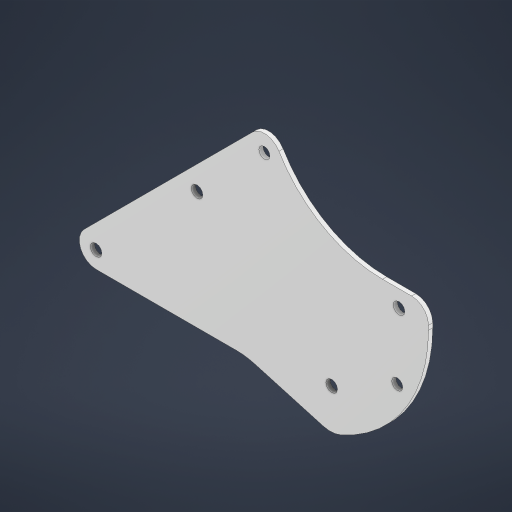
# Autodesk Inventor part: sled
Saved by Autodesk Inventor 2024 (Build 280153000, 153)
## iProperties
Created: 2023-08-16
Part Number: sled
Material: Acetal Resin, White
Document SubType Name: Modeling
Designer: avere
Density: 1.425 g/cm^3
Appearance: Smooth - White
Author: avere
Autodesk Inventor part; units mm, degrees
ref_plane "YZ Plane" through (0, 0, 0) normal (1, 0, 0) x (0, 1, 0)
ref_plane "XZ Plane" through (0, 0, 0) normal (0, 1, 0) x (-1, 0, 0)
ref_plane "XY Plane" through (0, 0, 0) normal (0, 0, 1) x (1, 0, 0)
sketch "Sketch1" plane through (0, 0, 0) normal (0, 0, 1) x (1, 0, 0)
  circle A0 centre (-18.3721, 25.1477) radius 2.1844
  circle A1 centre (57.8279, 25.1477) radius 2.1844
  circle A2 centre (32.4279, -12.9523) radius 2.1844
  circle A3 centre (-56.4721, -12.9523) radius 2.1844
  arc A4 (-60.9623, -8.4622) -> (-56.4721, -19.3023) centre (-56.4721, -12.9523) ccw
  arc A5 (-18.3721, 31.4977) -> (-22.8623, 29.6378) centre (-18.3721, 25.1477) ccw
  line L0 (68.9404, 23.5133) -> (68.9404, 25.1477)
  line L1 (62.5904, 31.4977) -> (57.8279, 31.4977)
  arc A6 (68.9404, 25.1477) -> (62.5904, 31.4977) centre (62.5904, 25.1477) ccw
  line L2 (-3.5614, -19.3023) -> (-56.4721, -19.3023)
  line L3 (-60.9623, -8.4622) -> (-22.8623, 29.6378)
  line L4 (-18.3721, 31.4977) -> (57.8279, 31.4977)
  arc A7 (35.7428, -27.2531) -> (68.9404, 23.5133) centre (13.525, 23.5133) ccw
  line L5 (29.3044, -27.6849) -> (3.4241, -20.2818)
  arc A8 (29.3044, -27.6849) -> (35.7428, -27.2531) centre (31.9239, -18.5272) ccw
  arc A9 (3.4241, -20.2818) -> (-3.5614, -19.3023) centre (-3.5614, -44.7023) ccw
  point P0 (0, 0)
  point P1 (32.4279, -28.5784)
  dimension "d0" = 4.3688
  dimension "d1" = 12.7
  dimension "d2" = 12.7
  dimension "d4" = 6.35
  dimension "d21" = 9.525
  dimension "d22" = 25.4
  constraints: 13 point on circle, 12 end point, 10 centre point, 10 tangent, 2 coincident, 2 vertical, 1 horizontal, 1 point on line, 3 other
  measures "d0" diameter of A1
  measures "d1" diameter of A4
  measures "d2" diameter of A5
  measures "d4" radius of A6
  measures "d21" radius of A8
  measures "d22" radius of A9
extrude "Extrusion1" add sketch "Sketch1" along normal blind 1.5875
sketch "Sketch2" plane through (0, 0, 1.5875) normal (0, 0, 1) x (1, 0, 0)
  circle A0 centre (57.15, 0) radius 2.0828
  point P0 (0, 0)
  dimension "d7" = 4.1656
  constraints: 1 centre point
  measures "d7" diameter of A0
extrude "Extrusion2" cut sketch "Sketch2" against normal blind 1.5875
sketch "Sketch3" plane through (57.8279, 25.1477, 1.5875) normal (0, 0, 1) x (1, 0, 0)
  circle A0 centre (-50.8, 25.4) radius 2.0828
  arc A1 (-45.3375, 28.6378) -> (-55.2901, 29.8901) centre (-50.8, 25.4) ccw
  line L0 (-80.6901, 4.4901) -> (-55.2901, 29.8901)
  arc A2 (-76.2, 6.35) -> (-80.6901, 4.4901) centre (-76.2, 0) ccw projected
  arc A3 (-45.3375, 28.6378) -> (-6.2178, 6.35) centre (-6.2178, 51.8254) ccw
  line L1 (4.7625, 6.35) -> (-76.2, 6.35) projected
  dimension "d17" = 4.1656
  constraints: 5 point on circle, 4 tangent, 3 centre point, 2 end point, 1 coincident, 1 point on line, 1 other
  measures "d17" diameter of A0
extrude "Extrusion4" add sketch "Sketch3" against normal blind 1.5875
body "Solid1"
